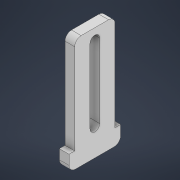
# Autodesk Inventor part: Ga mica 5mm
Saved by Autodesk Inventor 2021 (Build 250183000, 183)
## iProperties
Created: 2022-11-16
Part Number: Ga mica 5mm
Material: Generic
Document SubType Name: Modeling
Designer: phand
Density: 1 g/cm^3
Appearance: Default
Author: phand
Autodesk Inventor part; units mm, degrees
ref_plane "YZ Plane" through (0, 0, 0) normal (1, 0, 0) x (0, 1, 0)
ref_plane "XZ Plane" through (0, 0, 0) normal (0, 1, 0) x (-1, 0, 0)
ref_plane "XY Plane" through (0, 0, 0) normal (0, 0, 1) x (1, 0, 0)
sketch "Sketch1" plane through (0, 0, 0) normal (1, 0, 0) x (0, 1, 0)
  line L0 (17.5, 8) -> (-17.5, 8)
  line L1 (-17.5, 8) -> (-17.5, -8)
  line L2 (-17.5, -8) -> (17.5, -8)
  line L3 (17.5, -8) -> (17.5, 8)
  line L4 (17.5, 8) -> (-17.5, -8) construction
  line L5 (-17.5, 8) -> (17.5, -8) construction
  point P0 (0, 0)
  dimension "d0" = 35
  dimension "d1" = 16
  constraints: 12 end point, 2 midpoint, 2 parallel, 1 horizontal, 1 perpendicular
  measures "d0" distance of L2.end L1.end
  measures "d1" distance of L1.end L0.end
extrude "Extrusion1" add sketch "Sketch1" along normal blind 3
sketch "Sketch2" plane through (3, 0, 0) normal (1, 0, 0) x (0, 0, -1)
  line L0 (-8, 17.5) -> (-8, -17.5) construction
  line L1 (-8, -12.5) -> (7.9898, -12.5) construction
  line L2 (-8, -17.5) -> (8, -17.5) construction
  line L3 (8, 17.5) -> (-8, 17.5) construction
  line L4 (-8, 17.5) -> (7.9898, -12.5) construction
  line L5 (8, -17.5) -> (8, 17.5) construction
  line L6 (8, 17.5) -> (-8, -12.5) construction
  line L7 (0, 14) -> (0, -9) construction
  line L8 (-1.5, 14) -> (-1.5, -9)
  line L9 (1.5, -9) -> (1.5, 14)
  arc A0 (1.5, 14) -> (-1.5, 14) centre (0, 14) ccw
  arc A1 (-1.5, -9) -> (1.5, -9) centre (0, -9) ccw
  line L10 (6.25, -12.5) -> (8, -12.5)
  line L11 (8, -12.5) -> (8, 17.5)
  line L12 (8, 17.5) -> (6.25, 17.5)
  line L13 (6.25, 17.5) -> (6.25, -12.5)
  line L14 (-6.25, -12.5) -> (-8, -12.5)
  line L15 (-8, -12.5) -> (-8, 17.5)
  line L16 (-8, 17.5) -> (-6.25, 17.5)
  line L17 (-6.25, 17.5) -> (-6.25, -12.5)
  point P0 (0, 0)
  point P1 (0, 2.5)
  point P2 (-7.9898, -12.5)
  dimension "d4" = 5
  dimension "d5" = 3
  dimension "d6" = 23
  dimension "d9" = 6.25
  constraints: 30 end point, 4 point on circle, 4 tangent, 3 parallel, 3 symmetric about line, 2 centre point, 2 horizontal, 2 midpoint, 2 point on line, 1 perpendicular, 1 vertical
  measures "d4" distance between parallel lines of L2 L1
  measures "d5" diameter of A1
  measures "d6" distance of L9.start L9.end
  measures "d9" horizontal distance of point (0, 0) L10.start
extrude "Extrusion2" cut sketch "Sketch2" against normal through all
fillet "Fillet1" radius 2 4 edges at (1.5, 17.5, 6.25) (1.5, 17.5, -6.25) (1.5, -17.5, 8) (1.5, -17.5, -8)
body "Solid1"
